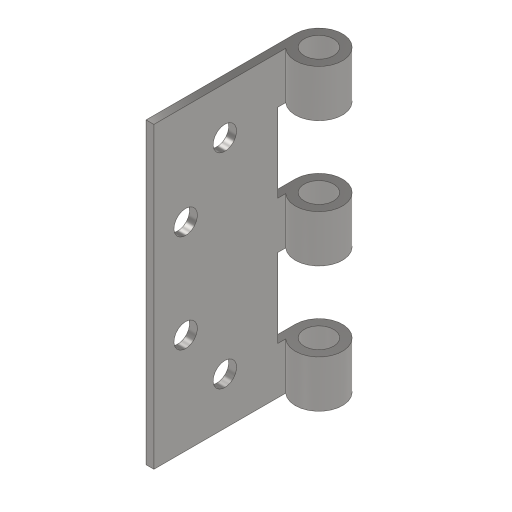
# Autodesk Inventor part: zawias-lewy
Saved by Autodesk Inventor 2023.2 (Build 272271000, 271)
## iProperties
Created: 2022-12-05
Part Number: zawias-lewy
Material: Stainless Steel
Document SubType Name: Modeling
Designer: GUT
Mass: 36.2804 g
Surface Area: 52.4704 cm^2
Volume: 4.53505 cm^3
Density: 8 g/cm^3
Appearance: Semi-Polished
Author: GUT
Autodesk Inventor part; units mm, degrees
ref_plane "YZ Plane" through (0, 0, 0) normal (1, 0, 0) x (0, 1, 0)
ref_plane "XZ Plane" through (0, 0, 0) normal (0, 1, 0) x (-1, 0, 0)
sketch "Sketch1" plane through (0, 0, 0) normal (1, 0, 0) x (0, 1, 0)
  line L0 (109.003, 50.5595) -> (32.803, 50.5595)
  line L1 (32.803, 50.5595) -> (32.803, 88.6595)
  line L2 (32.803, 88.6595) -> (109.003, 88.6595)
  line L3 (109.003, 88.6595) -> (109.003, 50.5595)
  line L4 (76.903, 50.5595) -> (97.003, 50.5595)
  line L5 (97.003, 50.5595) -> (97.003, 57.0595)
  line L6 (97.003, 57.0595) -> (76.903, 57.0595)
  line L7 (76.903, 57.0595) -> (76.903, 50.5595)
  line L8 (44.803, 50.5595) -> (64.903, 50.5595)
  line L9 (64.903, 50.5595) -> (64.903, 57.0595)
  line L10 (64.903, 57.0595) -> (44.803, 57.0595)
  line L11 (44.803, 57.0595) -> (44.803, 50.5595)
  circle A0 centre (97.003, 70.5595) radius 3
  circle A1 centre (83.403, 80.5595) radius 3
  line L12 (70.903, 88.6595) -> (70.903, 50.5595) construction
  circle A2 centre (44.803, 70.5595) radius 3
  circle A3 centre (58.403, 80.5595) radius 3
  point P0 (0, 0)
  dimension "d0" = 76.2
  dimension "d1" = 38.1
  dimension "d2" = 6.5
  dimension "d4" = 12
  dimension "d5" = 12
  dimension "d6" = 12
  dimension "d7" = 6
  dimension "d8" = 6
  dimension "d9" = 20
  dimension "d10" = 30
  dimension "d11" = 12.5
  dimension "d12" = 26.1
  constraints: 26 end point, 6 parallel, 4 centre point, 3 horizontal, 3 perpendicular, 2 equal length, 2 midpoint, 2 point on line, 2 symmetric about line, 2 other
  measures "d0" distance of L1.end L2.end
  measures "d1" distance of L0.end L1.end
  measures "d2" distance of L6.end L4.start
  measures "d4" distance between parallel lines of L3 L5
  measures "d5" distance between parallel lines of L1 L11
  measures "d6" distance between parallel lines of L9 L7
  measures "d7" diameter of A0
  measures "d8" diameter of A1
  measures "d9" distance from line of L0 A0.centre
  measures "d10" distance from line of L0 A1.centre
  measures "d11" distance from line of L12 A1.centre
  measures "d12" distance from line of L12 A0.centre
extrude "Extrusion1" add sketch "Sketch1" along normal blind 2 contours L0 L5 L6 L7 L9 L10 L11 L1 L2 L3
ref_plane "Work Plane1" through (2, 70.903, 50.5595) normal (0, 1, 0) x (-1, 0, 0)
sketch "Sketch2" plane through (0, 109.003, 88.6595) normal (0, 1, 0) x (1, 0, 0)
  line L0 (0, 38.1) -> (0, 0) projected
  line L1 (0, 0) -> (2, 0) projected
  line L2 (2, 38.1) -> (2, 0) projected
  line L3 (0, 38.1) -> (2, 38.1) projected
  circle A0 centre (6, 38.1) radius 6
  line L4 (0, 38.1) -> (2, 38.1) projected
  line L5 (0, 38.1) -> (2, 38.1)
  circle A1 centre (6, 38.1) radius 3.75
  point P0 (0, 88.6595)
  point P1 (1.2193, 34.4744)
  point P2 (0, 38.1)
  dimension "d15" = 0
  dimension "d16" = 12
  dimension "d18" = 7.5
  dimension "d23" = 4
  constraints: 2 centre point, 2 end point, 2 point on circle, 1 coincident
  measures "d15" distance from line of L3 A0.centre
  measures "d16" diameter of A0
  measures "d18" diameter of A1
  measures "d23" distance from line of L2 A0.centre
extrude "Extrusion2" add sketch "Sketch2" against normal up to surface (12 mm away) contours A0 L2 L3 | L3 L2 A0
mirror "Mirror1" about plane through (2, 70.903, 50.5595) normal (0, 1, 0) of "Extrusion2"
sketch "Sketch3" plane through (0, 76.903, 57.0595) normal (0, 1, 0) x (1, 0, 0)
  line L0 (0, -31.6) -> (2, -31.6) projected
  line L1 (0, 6.5) -> (2, 6.5) projected
  line L2 (0, 6.5) -> (2, 6.5)
  line L3 (0, 6.5) -> (0, -31.6) projected
  line L4 (2, 2.0279) -> (2, -31.6) projected
  arc A0 (2, 2.0279) -> (0, 6.5) centre (6, 6.5) ccw projected
  circle A1 centre (6, 6.5) radius 3.75 projected
  circle A2 centre (6, 6.5) radius 3.75 projected
  line L5 (0, 6.5) -> (0, -31.6) projected
  line L6 (0, -31.6) -> (2, -31.6) projected
  line L7 (2, 2.0279) -> (2, -31.6) projected
  arc A3 (2, 2.0279) -> (0, 6.5) centre (6, 6.5) ccw projected
  line L8 (2, 6.5) -> (2, 0) projected
  point P0 (0, 57.0595)
  constraints: 2 end point, 1 horizontal
extrude "Extrusion3" add sketch "Sketch3" against normal up to surface (12 mm away) contours A0 L8 L1
equation "\"d5\" = d4"
equation "\"d6\" = d4"
equation "\"d8\" = d7"
body "Solid1"
